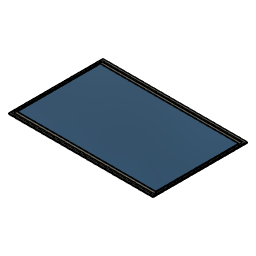
Proiect3D (Autodesk Fusion 360 archive; units mm, degrees)
design "Display"
Autodesk Fusion 360 part; units mm, degrees
sketch "Sketch1" plane through (0, 0, 0) normal (0, 0, 1) x (1, 0, 0)
  line L0 (85.1, 55.6) -> (-85.1, 55.6)
  line L1 (-85.1, 55.6) -> (-85.1, -55.6)
  line L2 (-85.1, -55.6) -> (85.1, -55.6)
  line L3 (85.1, -55.6) -> (85.1, 55.6)
  line L4 (85.1, 55.6) -> (-85.1, -55.6) construction
  line L5 (-85.1, 55.6) -> (85.1, -55.6) construction
  line L6 (83.9, 53.545) -> (-83.9, 53.545)
  line L7 (-83.9, 53.545) -> (-83.9, -53.545)
  line L8 (-83.9, -53.545) -> (83.9, -53.545)
  line L9 (83.9, -53.545) -> (83.9, 53.545)
  line L10 (83.9, 53.545) -> (-83.9, -53.545) construction
  line L11 (-83.9, 53.545) -> (83.9, -53.545) construction
  line L12 (82.4, 52.045) -> (-82.4, 52.045)
  line L13 (-82.4, 52.045) -> (-82.4, -52.045)
  line L14 (-82.4, -52.045) -> (82.4, -52.045)
  line L15 (82.4, -52.045) -> (82.4, 52.045)
  line L16 (82.4, 52.045) -> (-82.4, -52.045) construction
  line L17 (-82.4, 52.045) -> (82.4, -52.045) construction
  line L18 (81.6, 48.96) -> (-81.6, 48.96)
  line L19 (-81.6, 48.96) -> (-81.6, -48.96)
  line L20 (-81.6, -48.96) -> (81.6, -48.96)
  line L21 (81.6, -48.96) -> (81.6, 48.96)
  line L22 (81.6, 48.96) -> (-81.6, -48.96) construction
  line L23 (-81.6, 48.96) -> (81.6, -48.96) construction
  dimension "d1" = 170.2
  dimension "d2" = 111.2
  dimension "d3" = 167.8
  dimension "d4" = 107.09
  dimension "d5" = 164.8
  dimension "d6" = 104.09
  dimension "d7" = 163.2
  dimension "d8" = 97.92
  constraint horizontal L0
  constraint perpendicular L0 L1
  constraint parallel L0 L2
  constraint parallel L1 L3
  constraint coincident L4 origin
  constraint coincident L5 origin
  constraint horizontal L6
  constraint perpendicular L6 L7
  constraint parallel L6 L8
  constraint parallel L7 L9
  constraint coincident L10 origin
  constraint coincident L11 origin
  constraint horizontal L12
  constraint perpendicular L12 L13
  constraint parallel L12 L14
  constraint parallel L13 L15
  constraint coincident L16 origin
  constraint coincident L17 origin
  constraint horizontal L18
  constraint perpendicular L18 L19
  constraint parallel L18 L20
  constraint parallel L19 L21
  constraint coincident L22 origin
  constraint coincident L23 origin
  measures "d1" distance of L1.end L2.end
  measures "d2" distance of L0.end L1.end
  measures "d3" distance of L7.end L8.end
  measures "d4" distance of L6.end L7.end
  measures "d5" distance of L13.end L14.end
  measures "d6" distance of L12.end L13.end
  measures "d7" distance of L19.end L20.end
  measures "d8" distance of L18.end L19.end
extrude "Extrude1" add sketch "Sketch1" against normal blind 0.7 contours L0 L1 L2 L3 makes body 1
extrude "Extrude2" add sketch "Sketch1" against normal blind 0.5 contours L6 L7 L8 L9 bodies 1
extrude "Extrude3" add sketch "Sketch1" against normal blind 0.2 contours L12 L13 L14 L15 bodies 1
extrude "Extrude4" add sketch "Sketch1" along normal blind 0.1 separate body contours L18 L19 L20 L21 makes body 2
extrude "Extrude5" add 1 faces at (27.2, -53.3867, 0) along direction (0, 0, -1) blind 1 separate body on bodies 1 makes body 3
